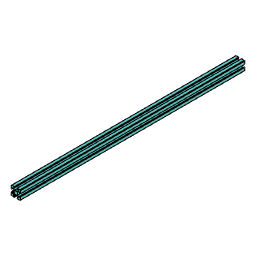
profile (Autodesk Fusion 360 design; units mm, degrees)
Autodesk Fusion 360 part; units mm, degrees
sketch "Sketch1" plane through (0, 0, 0) normal (0, 1, 0) x (1, 0, 0)
  line L0 (3.5, 0) -> (3.5, -2.7929)
  line L1 (3.5, -2.7929) -> (5.7071, -5)
  line L2 (5.7071, -5) -> (8, -5)
  line L3 (10, -3) -> (10, -10)
  line L4 (0, 0) -> (10, -10)
  line L5 (3.5, 0) -> (0, 0)
  line L6 (8, -5) -> (8, -3)
  line L7 (8, -3) -> (10, -3)
  dimension "d4" = 45
  dimension "d5" = 0.5
  dimension "d7" = 7
  dimension "d8" = 2
  dimension "d9" = 2
  dimension "d10" = 3.5
  dimension "d11" = 10
  constraint vertical L0
  constraint perpendicular L0 L2
  constraint perpendicular L2 L3
  constraint coincident L4.start L5.end
  constraint perpendicular L0 L5
  constraint parallel L1 L4
  constraint perpendicular L2 L6
  constraint horizontal L7
  measures "d4" angle of L4 L5
  measures "d5" distance of L1 L4
  measures "d7" distance of L3.start L3.end
  measures "d8" distance of L2.end L6.end
  measures "d9" distance of L3.start L6.end
  measures "d10" distance of L0.start L4.start
  measures "d11" distance of L4.start L3
extrude "Extrude1" add sketch "Sketch1" along normal blind 490
mirror "Mirror1" about plane through (0, 0, 0) normal (-0.707107, 0, 0.707107) of bodies 1 merged
mirror "Mirror2" about plane through (0, 0, 3.5) normal (-1, 0, 0) of bodies 1 merged
mirror "Mirror3" about plane through (3.5, 0, 0) normal (0, 0, -1) of bodies 1 merged
fillet "Fillet1" radius 1 4 edges at (-10, 245, 10) (10, 245, 10) (-10, 245, -10) (10, 245, -10)
sketch "Sketch2" plane through (0, 0, 0) normal (0, -1, 0) x (1, 0, 0)
  arc A0 (9, -10) -> (10, -9) centre (9, -9) ccw
  line L0 (10, -9) -> (10, -3)
  line L1 (10, -3) -> (8, -3)
  line L2 (8, -3) -> (8, -5)
  line L3 (8, -5) -> (5.7071, -5)
  line L4 (5.7071, -5) -> (3.5, -2.7929)
  line L5 (3.5, -2.7929) -> (3.5, 2.7929)
  line L6 (3.5, 2.7929) -> (5.7071, 5)
  line L7 (5.7071, 5) -> (8, 5)
  line L8 (8, 5) -> (8, 3)
  line L9 (8, 3) -> (10, 3)
  line L10 (10, 3) -> (10, 9)
  arc A1 (10, 9) -> (9, 10) centre (9, 9) ccw
  line L11 (9, 10) -> (3, 10)
  line L12 (3, 10) -> (3, 8)
  line L13 (3, 8) -> (5, 8)
  line L14 (5, 8) -> (5, 5.7071)
  line L15 (5, 5.7071) -> (2.7929, 3.5)
  line L16 (2.7929, 3.5) -> (-2.7929, 3.5)
  line L17 (-2.7929, 3.5) -> (-5, 5.7071)
  line L18 (-5, 5.7071) -> (-5, 8)
  line L19 (-5, 8) -> (-3, 8)
  line L20 (-3, 8) -> (-3, 10)
  line L21 (-3, 10) -> (-9, 10)
  arc A2 (-9, 10) -> (-10, 9) centre (-9, 9) ccw
  line L22 (-10, 9) -> (-10, 3)
  line L23 (-10, 3) -> (-8, 3)
  line L24 (-8, 3) -> (-8, 5)
  line L25 (-8, 5) -> (-5.7071, 5)
  line L26 (-5.7071, 5) -> (-3.5, 2.7929)
  line L27 (-3.5, 2.7929) -> (-3.5, -2.7929)
  line L28 (-3.5, -2.7929) -> (-5.7071, -5)
  line L29 (-5.7071, -5) -> (-8, -5)
  line L30 (-8, -5) -> (-8, -3)
  line L31 (-8, -3) -> (-10, -3)
  line L32 (-10, -3) -> (-10, -9)
  arc A3 (-10, -9) -> (-9, -10) centre (-9, -9) ccw
  line L33 (-9, -10) -> (-3, -10)
  line L34 (-3, -10) -> (-3, -8)
  line L35 (-3, -8) -> (-5, -8)
  line L36 (-5, -8) -> (-5, -5.7071)
  line L37 (-5, -5.7071) -> (-2.7929, -3.5)
  line L38 (-2.7929, -3.5) -> (2.7929, -3.5)
  line L39 (2.7929, -3.5) -> (5, -5.7071)
  line L40 (5, -5.7071) -> (5, -8)
  line L41 (5, -8) -> (3, -8)
  line L42 (3, -8) -> (3, -10)
  line L43 (3, -10) -> (9, -10)
  line L44 (2.9, 7.9) -> (4.9, 7.9)
  line L45 (4.9, 7.9) -> (4.9, 5.7485)
  line L46 (4.9, 5.7485) -> (2.7515, 3.6)
  line L47 (2.7515, 3.6) -> (-2.7515, 3.6)
  line L48 (-2.7515, 3.6) -> (-4.9, 5.7485)
  line L49 (-4.9, 5.7485) -> (-4.9, 7.9)
  line L50 (-4.9, 7.9) -> (-2.9, 7.9)
  line L51 (-2.9, 7.9) -> (-2.9, 10.1)
  line L52 (-2.9, 10.1) -> (-9, 10.1)
  arc A4 (-9, 10.1) -> (-10.1, 9) centre (-9, 9) ccw
  line L53 (-10.1, 9) -> (-10.1, 2.9)
  line L54 (-10.1, 2.9) -> (-7.9, 2.9)
  line L55 (-7.9, 2.9) -> (-7.9, 4.9)
  line L56 (-7.9, 4.9) -> (-5.7485, 4.9)
  line L57 (-5.7485, 4.9) -> (-3.6, 2.7515)
  line L58 (-3.6, 2.7515) -> (-3.6, -2.7515)
  line L59 (-3.6, -2.7515) -> (-5.7485, -4.9)
  line L60 (-5.7485, -4.9) -> (-7.9, -4.9)
  line L61 (-7.9, -4.9) -> (-7.9, -2.9)
  line L62 (-7.9, -2.9) -> (-10.1, -2.9)
  line L63 (-10.1, -2.9) -> (-10.1, -9)
  arc A5 (-10.1, -9) -> (-9, -10.1) centre (-9, -9) ccw
  line L64 (-9, -10.1) -> (-2.9, -10.1)
  line L65 (-2.9, -10.1) -> (-2.9, -7.9)
  line L66 (-2.9, -7.9) -> (-4.9, -7.9)
  line L67 (-4.9, -7.9) -> (-4.9, -5.7485)
  line L68 (-4.9, -5.7485) -> (-2.7515, -3.6)
  line L69 (-2.7515, -3.6) -> (2.7515, -3.6)
  line L70 (2.7515, -3.6) -> (4.9, -5.7485)
  line L71 (4.9, -5.7485) -> (4.9, -7.9)
  line L72 (4.9, -7.9) -> (2.9, -7.9)
  line L73 (2.9, -7.9) -> (2.9, -10.1)
  line L74 (2.9, -10.1) -> (9, -10.1)
  arc A6 (9, -10.1) -> (10.1, -9) centre (9, -9) ccw
  line L75 (10.1, -9) -> (10.1, -2.9)
  line L76 (10.1, -2.9) -> (7.9, -2.9)
  line L77 (7.9, -2.9) -> (7.9, -4.9)
  line L78 (7.9, -4.9) -> (5.7485, -4.9)
  line L79 (5.7485, -4.9) -> (3.6, -2.7515)
  line L80 (3.6, -2.7515) -> (3.6, 2.7515)
  line L81 (3.6, 2.7515) -> (5.7485, 4.9)
  line L82 (5.7485, 4.9) -> (7.9, 4.9)
  line L83 (7.9, 4.9) -> (7.9, 2.9)
  line L84 (7.9, 2.9) -> (10.1, 2.9)
  line L85 (10.1, 2.9) -> (10.1, 9)
  arc A7 (10.1, 9) -> (9, 10.1) centre (9, 9) ccw
  line L86 (9, 10.1) -> (2.9, 10.1)
  line L87 (2.9, 10.1) -> (2.9, 7.9)
  dimension "d22" = 0.1
sketch "Sketch3" plane through (0, 0, 0) normal (0, 1, 0) x (1, 0, 0)
  line L0 (10.1, 9) -> (10.1, 2.9)
  arc A0 (10.1, 9) -> (9, 10.1) centre (9, 9) ccw
  line L1 (2.9, 10.1) -> (9, 10.1)
  line L2 (2.9, 7.9) -> (2.9, 10.1)
  line L3 (4.9, 7.9) -> (2.9, 7.9)
  line L4 (4.9, 5.7485) -> (4.9, 7.9)
  line L5 (2.7515, 3.6) -> (4.9, 5.7485)
  line L6 (5.7485, 4.9) -> (3.6, 2.7515)
  line L7 (7.9, 4.9) -> (5.7485, 4.9)
  line L8 (7.9, 2.9) -> (7.9, 4.9)
  line L9 (10.1, 2.9) -> (7.9, 2.9)
  line L10 (3.6, 2.7515) -> (3.6, -2.7515)
  line L11 (3.6, -2.7515) -> (5.7485, -4.9)
  line L12 (5.7485, -4.9) -> (7.9, -4.9)
  line L13 (7.9, -4.9) -> (7.9, -2.9)
  line L14 (7.9, -2.9) -> (10.1, -2.9)
  line L15 (10.1, -2.9) -> (10.1, -9)
  arc A1 (9, -10.1) -> (10.1, -9) centre (9, -9) ccw
  line L16 (9, -10.1) -> (2.9, -10.1)
  line L17 (2.9, -10.1) -> (2.9, -7.9)
  line L18 (2.9, -7.9) -> (4.9, -7.9)
  line L19 (4.9, -7.9) -> (4.9, -5.7485)
  line L20 (4.9, -5.7485) -> (2.7515, -3.6)
  line L21 (2.7515, -3.6) -> (-2.7515, -3.6)
  line L22 (-2.7515, -3.6) -> (-4.9, -5.7485)
  line L23 (-4.9, -5.7485) -> (-4.9, -7.9)
  line L24 (-4.9, -7.9) -> (-2.9, -7.9)
  line L25 (-2.9, -7.9) -> (-2.9, -10.1)
  line L26 (-2.9, -10.1) -> (-9, -10.1)
  arc A2 (-10.1, -9) -> (-9, -10.1) centre (-9, -9) ccw
  line L27 (-10.1, -9) -> (-10.1, -2.9)
  line L28 (-10.1, -2.9) -> (-7.9, -2.9)
  line L29 (-7.9, -2.9) -> (-7.9, -4.9)
  line L30 (-7.9, -4.9) -> (-5.7485, -4.9)
  line L31 (-5.7485, -4.9) -> (-3.6, -2.7515)
  line L32 (-3.6, -2.7515) -> (-3.6, 2.7515)
  line L33 (-3.6, 2.7515) -> (-5.7485, 4.9)
  line L34 (-7.9, 2.9) -> (-10.1, 2.9)
  line L35 (-7.9, 4.9) -> (-7.9, 2.9)
  line L36 (-5.7485, 4.9) -> (-7.9, 4.9)
  line L37 (-10.1, 2.9) -> (-10.1, 9)
  line L38 (-4.9, 5.7485) -> (-2.7515, 3.6)
  line L39 (-2.7515, 3.6) -> (2.7515, 3.6)
  line L40 (-4.9, 7.9) -> (-4.9, 5.7485)
  line L41 (-2.9, 7.9) -> (-4.9, 7.9)
  line L42 (-2.9, 10.1) -> (-2.9, 7.9)
  line L43 (-9, 10.1) -> (-2.9, 10.1)
  arc A3 (-9, 10.1) -> (-10.1, 9) centre (-9, 9) ccw
